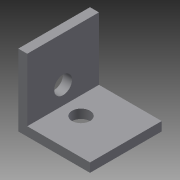
# Autodesk Inventor part: Other corner
Saved by Autodesk Inventor 2014 (Build 180170000, 170)
## iProperties
Created: 2014-01-06
Part Number: Other corner
Material: Generic
Document SubType Name: Modeling
Designer: Tristan Debrunner
Density: 1 g/cm^3
Appearance: Default
Mass: 3.63962 g
Surface Area: 28.8306 cm^2
Volume: 3.63962 cm^3
Author: Tristan Debrunner
Autodesk Inventor part; units mm, degrees
ref_plane "YZ Plane" through (0, 0, 0) normal (1, 0, 0) x (0, 1, 0)
ref_plane "XZ Plane" through (0, 0, 0) normal (0, 1, 0) x (-1, 0, 0)
ref_plane "XY Plane" through (0, 0, 0) normal (0, 0, 1) x (1, 0, 0)
sketch "Sketch1" plane through (0, 0, 0) normal (0, 0, 1) x (1, 0, 0)
  line L0 (0, 0) -> (25.4, 0)
  line L1 (25.4, 0) -> (25.4, 3.175)
  line L2 (25.4, 3.175) -> (3.175, 3.175)
  line L3 (3.175, 3.175) -> (3.175, 25.4)
  line L4 (3.175, 25.4) -> (0, 25.4)
  line L5 (0, 25.4) -> (0, 0)
  dimension "d0" = 25.4
  dimension "d1" = 3.175
  dimension "d2" = 22.225
  dimension "d3" = 22.225
  dimension "d4" = 3.175
  constraints: 12 end point, 3 perpendicular, 1 horizontal, 1 parallel
  measures "d0" distance of L0.start L0.end
  measures "d1" distance of L0.end L1.end
  measures "d2" distance of L1.end L2.end
  measures "d3" distance of L2.end L3.end
  measures "d4" distance of L3.end L4.end
extrude "Extrusion1" add sketch "Sketch1" along normal blind 25.4
sketch "Sketch2" plane through (0, 0, 0) normal (0, -1, 0) x (1, 0, 0)
  line L0 (0, 0) -> (0, 25.4) projected
  line L1 (0, 12.7) -> (9.525, 12.7)
  dimension "d7" = 9.525
  constraints: 2 end point, 1 midpoint, 1 perpendicular
  measures "d7" distance of L1.start L1.end
hole "Hole1" at (9.525, 0, 12.7) direction (0, 1, 0) diameter 6.35 end through all
sketch "Sketch3" plane through (0, 0, 0) normal (-1, 0, 0) x (0, 0, 1)
  line L0 (0, 0) -> (25.4, 0) projected
  line L1 (0, 25.4) -> (25.4, 25.4) projected
  line L2 (12.7, 0) -> (12.7, 9.525)
  dimension "d15" = 9.525
  constraints: 2 end point, 1 midpoint, 1 perpendicular
  measures "d15" distance of L2.start L2.end
hole "Hole2" at (0, 9.525, 12.7) direction (1, 0, 0) diameter 6.35 end through all
body "Solid1"
